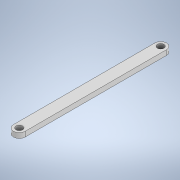
# Autodesk Inventor part: tay quay
Saved by Autodesk Inventor 2020 (Build 240168000, 168)
## iProperties
Created: 2022-11-23
Part Number: tay quay
Material: Generic
Document SubType Name: Modeling
Designer: ADMIN
Density: 1 g/cm^3
Appearance: Default
Author: ADMIN
Autodesk Inventor part; units mm, degrees
ref_plane "YZ Plane" through (0, 0, 0) normal (1, 0, 0) x (0, 1, 0)
ref_plane "XZ Plane" through (0, 0, 0) normal (0, 1, 0) x (-1, 0, 0)
ref_plane "XY Plane" through (0, 0, 0) normal (0, 0, 1) x (1, 0, 0)
sketch "Sketch1" plane through (0, 0, 0) normal (0, 1, 0) x (-1, 0, 0)
  arc A0 (3.5, 0) -> (-3.5, 0) centre (0, 0) ccw
  arc A1 (-3.5, -85) -> (3.5, -85) centre (0, -85) ccw
  line L0 (3.5, 0) -> (3.5, -85)
  line L1 (-3.5, 0) -> (-3.5, -85)
  dimension "d0" = 7
  dimension "d1" = 7
  dimension "d9" = 85
  constraints: 4 end point, 4 point on circle, 2 centre point, 1 coincident, 1 parallel, 1 tangent, 1 vertical
  measures "d0" diameter of A0
  measures "d1" diameter of A1
  measures "d9" distance of L1.start L1.end
extrude "Extrusion1" add sketch "Sketch1" along normal blind 3
sketch "Sketch2" plane through (0, 3, 0) normal (0, 1, 0) x (1, 0, 0)
  circle A0 centre (0, 0) radius 2
  circle A1 centre (0, 85) radius 2
  arc A2 (3.5, 85) -> (-3.5, 85) centre (0, 85) ccw projected
  dimension "d4" = 4
  dimension "d5" = 4
  dimension "d10" = 1.5
  constraints: 2 centre point, 1 coincident
  measures "d4" diameter of A0
  measures "d5" diameter of A1
  measures "d10" radial gap between concentric circles of A1 A2
extrude "Extrusion2" cut sketch "Sketch2" against normal blind 3
body "Solid1"
